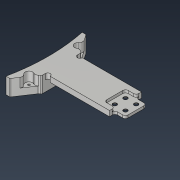
# Autodesk Inventor part: Kicker Sichel
Saved by Autodesk Inventor 2022.1 (Build 261234020, 234B)
## iProperties
Part Number: Kicker Sichel
Material: Aluminium 6061
Document SubType Name: Modeling
Designer: rYan
Mass: 26.3222 g
Surface Area: 53.2988 cm^2
Volume: 9.74896 cm^3
Density: 2.7 g/cm^3
Appearance: Aluminium - flach
Author: rYan
Autodesk Inventor part; units mm, degrees
ref_plane "YZ Plane" through (0, 0, 0) normal (1, 0, 0) x (0, 1, 0)
ref_plane "XZ Plane" through (0, 0, 0) normal (0, 1, 0) x (-1, 0, 0)
ref_plane "XY Plane" through (0, 0, 0) normal (0, 0, 1) x (1, 0, 0)
sketch "Skizze1" plane through (0, 0, 0) normal (0, 0, 1) x (1, 0, 0)
  line L0 (3.6, 12) -> (48, 12)
  line L1 (48, 12) -> (48, -12)
  line L2 (48, -12) -> (3.6, -12)
  line L3 (-189.6, 0) -> (87.6, 0) projected
  line L4 (-1, 15) -> (-10, 28.5)
  line L5 (-1, -15) -> (-10, -28.5)
  line L6 (-10, -28.5) -> (-12.9316, -28.5)
  line L7 (-10, 28.5) -> (-12.9316, 28.5)
  arc A0 (-12.9316, -28.5) -> (-12.9316, 28.5) centre (-150, 0) ccw
  line L8 (-10, 28.5) -> (-10, -28.5) construction
  line L9 (0, 39.9) -> (0, -39.9) projected
  line L10 (-2, 12.5) -> (-2, -9.8115) construction
  arc A1 (0, 12) -> (3.6, 12) centre (1.8, 12) ccw
  arc A2 (3.6, -12) -> (0, -12) centre (1.8, -12) ccw
  line L11 (0, 12) -> (0, 15)
  line L12 (0, 15) -> (-1, 15)
  line L13 (0, -12) -> (0, -15)
  line L14 (0, -15) -> (-1, -15)
  point P0 (0, 0)
  dimension "d2" = 24
  dimension "d52" = 140
  dimension "d55" = 57
  dimension "d59" = 8
  dimension "d60" = 2
  dimension "d64" = 0
  dimension "d73" = 1.8
  dimension "d75" = 48
  dimension "d76" = 30
  dimension "d77" = 1
  constraints: 26 end point, 7 point on line, 6 point on circle, 3 centre point, 3 horizontal, 3 perpendicular, 3 vertical, 2 parallel, 1 line through centre, 1 tangent, 6 other
  measures "d2" distance of L0.end L1.end
  measures "d52" radius of A0
  measures "d55" distance between parallel lines of L6 L7
  measures "d60" distance between parallel lines of L9 L10
  measures "d64" horizontal distance of L8 L4.end
  measures "d73" radius of A1
  measures "d75" distance between parallel lines of L1 L9
  measures "d76" distance between parallel lines of L14 L12
  measures "d77" distance of L11.end L4.start
extrude "Extrusion1" add sketch "Skizze1" along normal blind 12
sketch "Skizze8" plane through (0, 0, 12) normal (0, 0, 1) x (1, 0, 0)
  line L0 (-189.6, 0) -> (87.6, 0) projected
  arc A0 (-12.9316, -28.5) -> (-12.9316, 28.5) centre (-150, 0) ccw projected
  line L1 (-1, 15) -> (-10, 28.5) projected
  line L2 (-11.2277, 18.5) -> (-3.3333, 18.5) construction
  point P0 (0, 0)
  point P1 (-5.7805, 18.5)
  point P2 (-5.7805, -18.5)
  point P3 (-11.6616, -21.5053)
  point P4 (-7.2805, 18.5)
  dimension "d65" = 18.5
  dimension "d80" = 1.5
  constraints: 2 end point, 2 point on line, 1 horizontal, 1 midpoint, 1 point on circle, 1 symmetric about line
  measures "d65" distance between parallel lines of L0 L2
  measures "d80" distance of point (-7.281, 18.5) point (-5.781, 18.5)
hole "Bohrung4" at (-5.7805, 18.5, 12) at (-5.7805, -18.5, 12) direction (0, 0, -1) diameter 1.567 end through all counterbore diameter 5.5 counterbore depth 7 thread size "M2x0.4" class "6H" standard "ISO Metric profile"
sketch "Skizze2" plane through (0, 0, 0) normal (0, 0, -1) x (-1, 0, 0)
  line L0 (-3.6, -12) -> (-48, -12) projected
  line L1 (-48, -12) -> (-48, 12) projected
  line L2 (-48, 12) -> (-3.6, 12) projected
  line L3 (0, -12) -> (-48, -12)
  line L4 (-48, -12) -> (-48, 12)
  line L5 (-48, 12) -> (0, 12)
  line L6 (-48, 12) -> (-3.6, 12) projected
  line L7 (0, 12) -> (0, -12)
  point P0 (0, 0)
  point P1 (0, -12.5)
  point P2 (0, 12.5)
  point P3 (-3.6, 12)
  constraints: 8 end point, 2 horizontal, 1 midpoint, 1 parallel, 1 perpendicular, 1 vertical, 4 other
extrude "Extrusion2" cut sketch "Skizze2" against normal blind 8
sketch "Skizze11" plane through (0, 0, 12) normal (0, 0, 1) x (1, 0, 0)
  line L0 (48, 12) -> (3.6, 12) construction
  line L1 (3.6, -12) -> (48, -12) construction
  line L2 (48, -12) -> (48, 12) construction
  line L3 (-25.1179, 0) -> (60.1863, 0) construction
  line L4 (48, -12) -> (48, 12) construction
  line L5 (48, 8) -> (42, 8)
  line L6 (40, 6) -> (40, -6)
  line L7 (42, -8) -> (48, -8)
  line L8 (48, -8) -> (48, 8)
  arc A0 (42, 8) -> (40, 6) centre (42, 6) ccw
  arc A1 (40, -6) -> (42, -8) centre (42, -6) ccw
  point P0 (0, 0)
  dimension "d109" = 2
  dimension "d110" = 8
  dimension "d111" = 4
  constraints: 8 end point, 4 point on circle, 4 tangent, 2 centre point, 2 parallel, 1 equal radius, 1 horizontal, 1 perpendicular, 1 point on line, 2 other
  measures "d109" radius of A0
  measures "d110" distance between parallel lines of L2 L6
  measures "d111" distance between parallel lines of L0 L5
extrude "Extrusion7" cut sketch "Skizze11" against normal blind 2
sketch "Skizze12" plane through (0, 0, 8) normal (0, 0, -1) x (-1, 0, 0)
  line L0 (-48, -12) -> (-48, 12) construction
  line L1 (-70.0434, 0) -> (26.7607, 0) construction
  line L2 (-48, -7.9) -> (-53.8, -7.9)
  line L3 (-55.8, -5.9) -> (-55.8, 5.9)
  line L4 (-53.8, 7.9) -> (-48, 7.9)
  line L5 (-48, 7.9) -> (-48, -7.9)
  arc A0 (-55.8, -5.9) -> (-53.8, -7.9) centre (-53.8, -5.9) ccw
  arc A1 (-53.8, 7.9) -> (-55.8, 5.9) centre (-53.8, 5.9) ccw
  point P0 (0, 0)
  dimension "d112" = 2
  dimension "d113" = 4.1
  dimension "d114" = 7.8
  constraints: 8 end point, 4 point on circle, 4 tangent, 2 centre point, 2 parallel, 1 equal radius, 1 horizontal, 1 perpendicular, 1 point on line, 2 other
  measures "d112" radius of A0
  measures "d113" distance from line of L0.start L2
  measures "d114" distance between parallel lines of L0 L3
extrude "Extrusion8" add sketch "Skizze12" against normal blind 2
sketch "Skizze13" plane through (0, 0, 8) normal (0, 0, -1) x (-1, 0, 0)
  line L0 (-64.9863, 0) -> (25.9179, 0) construction
  line L1 (0, -39.9) -> (0, 39.9) construction
  line L2 (-48, -12) -> (-48, -7.9) construction
  line L3 (-44, -4) -> (-52, -4) construction
  line L4 (-52, -4) -> (-52, 4) construction
  line L5 (-52, 4) -> (-44, 4) construction
  line L6 (-44, 4) -> (-44, -4) construction
  point P0 (0, 0)
  dimension "d118" = 8
  dimension "d119" = 8
  constraints: 8 end point, 4 coincident, 2 parallel, 1 horizontal, 1 perpendicular, 2 other
  measures "d118" distance of L3.start L3.end
  measures "d119" distance of L5.end L3.start
hole "Bohrung5" at (44, -4, 8) at (52, -4, 8) at (52, 4, 8) at (44, 4, 8) direction (0, 0, 1) diameter 3 end through all countersink diameter 6.7 countersink angle 90
fillet "Rundung6" radius 2 4 edges at (48, -8, 11) (48, -7.9, 9) (48, 8, 11) (48, 7.9, 9)
sketch "Skizze3" plane through (0, 0, 8) normal (0, 0, -1) x (-1, 0, 0)
  line L0 (-3.6, -12) -> (-48, -12) projected
  line L1 (-48, -12) -> (-48, 12) projected
  line L2 (-48, 12) -> (-3.6, 12) projected
  line L3 (-48, -12) -> (-44, -12)
  line L4 (-44, -12) -> (-44, 12)
  line L5 (-44, 12) -> (-48, 12)
  line L6 (-48, 12) -> (-48, -12)
  point P0 (0, 0)
  point P1 (0, -12.5)
  point P2 (0, 12.5)
  point P3 (10, -12.5)
  point P4 (-3.6, 12)
  dimension "d9" = 4
  constraints: 8 end point, 2 parallel, 1 horizontal, 1 perpendicular, 3 other
  measures "d9" distance between parallel lines of L1 L4
extrude "Extrusion3" [suppressed]
sketch "Skizze4" plane through (0, 0, 12) normal (0, 0, 1) x (1, 0, 0)
  line L0 (48, -12) -> (48, 12) projected
  line L1 (-25.1179, 0) -> (60.1863, 0) projected
  point P0 (0, 0)
  point P1 (46, 0)
  dimension "d12" = 2
  constraints: 1 point on line
  measures "d12" distance from line of L0 point (46, 0)
hole "Bohrung1" [suppressed]
pattern_linear "Rechteckige Anordnung1" [suppressed]
fillet "Rundung1" radius 2 2 edges at (-1, -15, 6) (-1, 15, 6)
fillet "Rundung2" radius 1 4 edges at (-10, -28.5, 6) (-10, 28.5, 6) (0, -15.0012, 6) (0, 15.0012, 6)
fillet "Rundung3" radius 2.5 4 edges at (-5.1116, -21.1674, 8.5) (-3.061, -18.0915, 8.5) (-5.1116, 21.1674, 8.5) (-3.061, 18.0915, 8.5)
